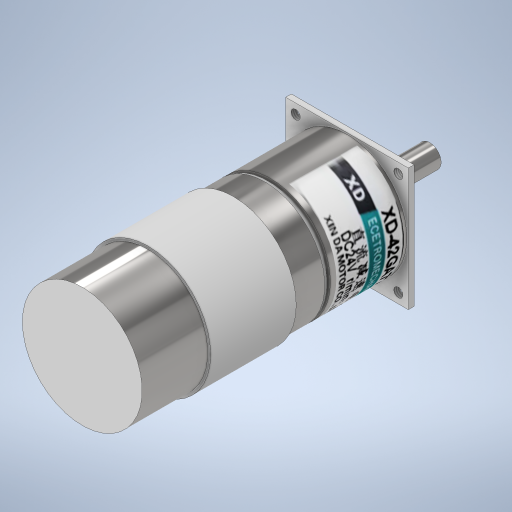
# Autodesk Inventor part: HCMUTE-CDT23-MOTOR_DC24V-100RPM-XD42GA775
Saved by Autodesk Inventor 2023 (Build 270158000, 158)
## iProperties
Created: 2023-10-11
Part Number: HCMUTE-CDT23-MOTOR_DC24V-100RPM-XD42GA775
Material: Generic
Document SubType Name: Modeling
Designer: havie
Density: 1 g/cm^3
Appearance: Default
Author: havie
Autodesk Inventor part; units mm, degrees
ref_plane "YZ Plane" through (0, 0, 0) normal (1, 0, 0) x (0, 1, 0)
ref_plane "XZ Plane" through (0, 0, 0) normal (0, 1, 0) x (-1, 0, 0)
sketch "Sketch1" plane through (0, 0, 0) normal (0, 1, 0) x (-1, 0, 0)
  circle A0 centre (0, 0) radius 21
  circle A1 centre (0, 0) radius 22
  dimension "d0" = 42
  dimension "d105" = 44
  constraints: 2 centre point, 2 coincident
  measures "d0" diameter of A0
  measures "d105" diameter of A1
extrude "Extrusion1" add sketch "Sketch1" along normal mid plane 66 contours A0
fillet "Fillet1" radius 2 1 edges at (21, 33, 0)
sketch "Sketch2" plane through (0, 33, 0) normal (0, 1, 0) x (1, 0, 0)
  circle A0 centre (0, 0) radius 21
  dimension "d4" = 42
  constraints: 1 centre point, 1 coincident
  measures "d4" diameter of A0
extrude "Extrusion2" add sketch "Sketch2" along normal blind 28.8
sketch "Sketch14" plane through (0, 61.8, 0) normal (0, 1, 0) x (1, 0, 0)
  line L0 (-21.5, 21.5) -> (21.5, 21.5)
  line L1 (21.5, 21.5) -> (21.5, -21.5)
  line L2 (21.5, -21.5) -> (-21.5, -21.5)
  line L3 (-21.5, -21.5) -> (-21.5, 21.5)
  line L4 (-21.5, 21.5) -> (21.5, -21.5) construction
  line L5 (21.5, 21.5) -> (-21.5, -21.5) construction
  point P0 (0, 0)
  dimension "d81" = 43
  dimension "d82" = 43
  constraints: 12 end point, 2 midpoint, 2 parallel, 1 horizontal, 1 perpendicular
  measures "d81" distance of L1.end L2.end
  measures "d82" distance of L0.end L1.end
extrude "Extrusion13" add sketch "Sketch14" against normal blind 2
sketch "Sketch15" plane through (0, 61.8, 0) normal (0, 1, 0) x (1, 0, 0)
  point P0 (0, 0)
  point P1 (-18, 18)
  point P2 (18, 18)
  point P3 (18, -18)
  point P4 (-18, -18)
  dimension "d85" = 36
  dimension "d86" = 36
  dimension "d87" = 18
  dimension "d88" = 18
  constraints: 2 horizontal alignment, 2 vertical alignment
  measures "d85" distance of point (-18, -18) point (-18, 18)
  measures "d86" distance of point (-18, 18) point (18, 18)
  measures "d87" horizontal distance of point (0, 0) point (18, 18)
  measures "d88" horizontal distance of point (0, 0) point (18, 18)
hole "Hole2" at (-18, 61.8, -18) at (18, 61.8, -18) at (18, 61.8, 18) at (-18, 61.8, 18) direction (0, -1, 0) diameter 3.242 end through all thread size "M4x0.7" class "6H" standard "ISO Metric profile"
sketch "Sketch16" plane through (0, 61.8, 0) normal (0, 1, 0) x (1, 0, 0)
  point P0 (0, 0)
sketch "Sketch17" plane through (0, 61.8, 0) normal (0, 1, 0) x (1, 0, 0)
  circle A0 centre (0, 0) radius 7
  dimension "d96" = 14
  constraints: 1 centre point, 1 coincident
  measures "d96" diameter of A0
extrude "Extrusion14" add sketch "Sketch17" along normal blind 7
sketch "Sketch18" plane through (0, 68.8, 0) normal (0, 1, 0) x (1, 0, 0)
  circle A0 centre (0, 0) radius 4
  dimension "d99" = 8
  constraints: 1 centre point, 1 coincident
  measures "d99" diameter of A0
extrude "Extrusion15" add sketch "Sketch18" along normal blind 20
sketch "Sketch19" plane through (0, 88.8, 0) normal (0, 1, 0) x (1, 0, 0)
  circle A0 centre (0, 0) radius 4 projected
  line L0 (-2.6458, 3) -> (2.6458, 3)
  dimension "d102" = 3
  constraints: 2 end point, 2 point on circle, 1 horizontal
  measures "d102" distance from line of point (0, 0) L0
extrude "Extrusion16" cut sketch "Sketch19" against normal blind 19 contours L0 A0 picked at (-0.6179, 3.1815)
extrude "Extrusion17" add sketch "Sketch1" along normal blind 20 and the other way blind 10
ref_plane "Work Plane3" through (21, 33, 0) normal (1, 0, 0) x (0, 0, -1)
sketch "Sketch20" plane through (21, 33, 0) normal (1, 0, 0) x (0, 0, -1)
  line L0 (20.5, 25.8) -> (20.5, 2.0287) construction
  line L1 (20.5, 2.0287) -> (-20.5, 2.0287) construction
  line L2 (-20.5, 2.0287) -> (-20.5, 25.8) construction
  line L3 (-20.5, 25.8) -> (20.5, 25.8) construction
  line L4 (21.5, 28.8) -> (21.5, 26.8) projected
  line L5 (-21.5, 28.8) -> (-21.5, 26.8) projected
  line L6 (21.5, 26.8) -> (-21.5, 26.8) projected
  point P0 (0, -33)
  dimension "d123" = 1
  dimension "d124" = 1
  dimension "d125" = 1
  constraints: 2 other
  measures "d123" distance between parallel lines of L4 L0
  measures "d124" distance between parallel lines of L5 L2
  measures "d125" distance between parallel lines of L6 L3
decal "Decal2"
body "Solid1"
